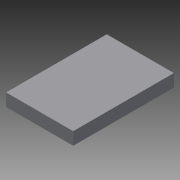
# Autodesk Inventor part: Motor Shim
Saved by Autodesk Inventor 2015 (Build 190159000, 159)
## iProperties
Created: 2016-03-22
Part Number: Motor Shim
Material: Generic
Document SubType Name: Modeling
Designer: Mac
Density: 1 g/cm^3
Appearance: Default
Author: Mac
Autodesk Inventor part; units mm, degrees
ref_plane "YZ Plane" through (0, 0, 0) normal (1, 0, 0) x (0, 1, 0)
ref_plane "XZ Plane" through (0, 0, 0) normal (0, 1, 0) x (-1, 0, 0)
ref_plane "XY Plane" through (0, 0, 0) normal (0, 0, 1) x (1, 0, 0)
sketch "Sketch2" plane through (0, 0, 0) normal (0, 1, 0) x (-1, 0, 0)
  line L0 (88.9, 76.2) -> (-88.9, 76.2)
  line L1 (-88.9, 76.2) -> (-88.9, -76.2)
  line L2 (-88.9, -76.2) -> (88.9, -76.2)
  line L3 (88.9, -76.2) -> (88.9, 76.2)
  point P0 (0, 0)
  point P1 (88.9, 0)
  point P2 (0, -76.2)
  dimension "d0" = 152.4
  dimension "d1" = 177.8
  constraints: 8 end point, 2 midpoint, 2 parallel, 1 horizontal, 1 horizontal alignment, 1 perpendicular, 1 vertical alignment
  measures "d0" distance of L2.end L0.start
  measures "d1" distance of L1.end L2.end
extrude "Extrusion1" add sketch "Sketch2" along normal blind 19.05
body "Solid1"
